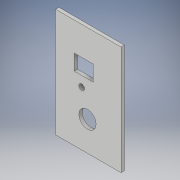
# Autodesk Inventor part: temp_sensor_back_plate
Saved by Autodesk Inventor 2018 (Build 220112000, 112)
## iProperties
Created: 2018-03-26
Part Number: temp_sensor_back_plate
Material: Generic
Document SubType Name: Modeling
Designer: Thomas
Density: 1 g/cm^3
Appearance: Default
Author: Thomas
Autodesk Inventor part; units mm, degrees
ref_plane "YZ Plane" through (0, 0, 0) normal (1, 0, 0) x (0, 1, 0)
ref_plane "XZ Plane" through (0, 0, 0) normal (0, 1, 0) x (-1, 0, 0)
ref_plane "XY Plane" through (0, 0, 0) normal (0, 0, 1) x (1, 0, 0)
sketch "Sketch1" plane through (20, 33.265, 0) normal (0, 0, 1) x (1, 0, 0)
  line L0 (0, 0) -> (-40, 0)
  line L1 (-40, 0) -> (-40, -66.53)
  line L2 (-40, -66.53) -> (0, -66.53)
  line L3 (0, -66.53) -> (0, 0)
  point P0 (-20, -33.265)
  dimension "d3" = 40
  dimension "d2" = 66.53
  dimension "d1" = 33.265
  dimension "d0" = 20
  constraints: 8 end point, 2 parallel, 1 horizontal, 1 perpendicular
  measures "d3" distance of L2.end L1.end
  measures "d2" distance between parallel lines of L2 L0
  measures "d1" distance from line of point (-20, -33.265) L2
  measures "d0" distance from line of L3 point (-20, -33.265)
extrude "Extrusion1" add sketch "Sketch1" along normal blind 2.04
sketch "Sketch2" plane through (0, 0, 0) normal (0, 0, 1) x (1, 0, 0)
  line L0 (2.95, 6.215) -> (-8.59, 6.215)
  line L1 (-8.59, 6.215) -> (-8.59, 15.765)
  line L2 (-8.59, 15.765) -> (2.95, 15.765)
  line L3 (2.95, 15.765) -> (2.95, 6.215)
  line L4 (20, -33.265) -> (20, 33.265) projected
  line L5 (20, 33.265) -> (-20, 33.265) projected
  circle A0 centre (-0.5, -15.215) radius 5.25
  line L6 (-20, 33.265) -> (-20, -33.265) projected
  line L7 (-20, -33.265) -> (20, -33.265) projected
  circle A1 centre (-4, 0.035) radius 1.75
  point P0 (0, 0)
  dimension "d7" = 17.05
  dimension "d8" = 11.54
  dimension "d9" = 9.55
  dimension "d10" = 17.5
  dimension "d11" = 19.5
  dimension "d12" = 10.5
  dimension "d13" = 18.05
  dimension "d14" = 16
  dimension "d15" = 3.5
  dimension "d16" = 33.3
  constraints: 8 end point, 2 centre point, 2 parallel, 1 horizontal, 1 perpendicular
  measures "d7" distance between parallel lines of L3 L4
  measures "d8" distance between parallel lines of L1 L3
  measures "d9" distance between parallel lines of L2 L0
  measures "d10" distance between parallel lines of L5 L2
  measures "d11" distance from line of L6 A0.centre
  measures "d12" diameter of A0
  measures "d13" distance from line of L7 A0.centre
  measures "d14" distance from line of L6 A1.centre
  measures "d15" diameter of A1
  measures "d16" distance from line of L7 A1.centre
extrude "Extrusion2" cut sketch "Sketch2" along normal up to next contours L0 L1 L2 L3 | A0 | A1
equation "\"d1\" = 0.5 * d2"
equation "\"d0\" = 0.5 * d3"
body "Solid1"
